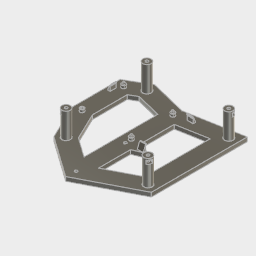
MPCNC Case 3 (Autodesk Fusion 360 design; units mm, degrees)
Autodesk Fusion 360 part; units mm, degrees
sketch "RAMBo" plane through (0, 0, 0) normal (0, 0, 1) x (1, 0, 0)
  line L0 (30.8759, -26.1352) -> (135.0159, -26.1352)
  line L1 (135.0159, -26.1352) -> (135.0159, 76.7348)
  line L2 (135.0159, 76.7348) -> (30.8759, 76.7348)
  line L3 (30.8759, 76.7348) -> (30.8759, -26.1352)
  line L4 (30.8759, 76.7348) -> (34.6859, 76.7348)
  line L5 (34.6859, 76.7348) -> (34.6859, 72.9248) construction
  line L6 (34.6859, 72.9248) -> (30.8759, 72.9248) construction
  line L7 (30.8759, 72.9248) -> (30.8759, 76.7348)
  line L8 (34.6859, 72.9248) -> (34.6859, -22.3252) construction
  line L9 (34.6859, -22.3252) -> (131.2059, -22.3252) construction
  line L10 (34.6859, 72.9248) -> (131.2059, 72.9248) construction
  circle A0 centre (34.6859, 72.9248) radius 1.625
  circle A1 centre (131.2059, 72.9248) radius 1.625
  circle A2 centre (34.6859, -22.3252) radius 1.625
  circle A3 centre (131.2059, -22.3252) radius 1.625
  line L11 (135.0159, -26.1352) -> (135.0159, 31.2053)
  line L12 (135.0159, -26.1352) -> (135.0159, 63.7808)
  line L13 (135.0159, 31.2053) -> (136.5659, 31.2053)
  line L14 (136.5659, 31.2053) -> (136.5659, 63.7808)
  line L15 (136.5659, 63.7808) -> (135.0159, 63.7808)
  line L16 (135.0159, 63.7808) -> (135.0159, 31.2053)
  line L17 (30.8759, -26.1352) -> (30.8759, 26.2523)
  line L18 (30.8759, -26.1352) -> (30.8759, 38.2538)
  line L19 (30.8759, 26.2523) -> (27.1959, 26.2523)
  line L20 (27.1959, 26.2523) -> (27.1959, 38.2538)
  line L21 (27.1959, 38.2538) -> (30.8759, 38.2538)
  line L22 (30.8759, 38.2538) -> (30.8759, 26.2523)
  dimension "d2" = 104.14
  dimension "d3" = 102.87
  dimension "d4" = 3.81
  dimension "d5" = 3.81
  dimension "d6" = 95.25
  dimension "d7" = 96.52
  dimension "d8" = 96.52
  dimension "d10" = 3.25
  dimension "d11" = 3.25
  dimension "d12" = 3.25
  dimension "d13" = 3.25
  dimension "d14" = 57.3405
  dimension "d15" = 89.916
  dimension "d16" = 1.55
  dimension "d17" = 52.3875
  dimension "d18" = 64.389
  dimension "d19" = 3.68
  measures "d2" distance of L0.start L0.end
  measures "d3" distance of L0.start L2.end
  measures "d4" distance of L2.end L6.end
  measures "d5" distance of L2.end L4.end
  measures "d6" distance of L5.end L8.end
  measures "d7" distance of L8.end L9.end
  measures "d8" distance of L5.end L10.end
  measures "d10" diameter of A0
  measures "d11" diameter of A1
  measures "d12" diameter of A2
  measures "d13" diameter of A3
  measures "d14" distance of L0.end L11.end
  measures "d15" distance of L0.end L12.end
  measures "d16" distance of L11.end L13.end
  measures "d17" distance of L0.start L17.end
  measures "d18" distance of L0.start L18.end
  measures "d19" distance of L17.end L19.end
sketch "RPi" plane through (0, 0, 0) normal (0, 0, 1) x (1, 0, 0)
  line L0 (17.3453, 10.3376) -> (17.3453, 13.8376) construction
  line L1 (17.3453, 13.8376) -> (13.8453, 13.8376) construction
  line L2 (16.8453, 10.3376) -> (16.8453, 13.3376) construction
  line L3 (16.8453, 13.3376) -> (13.8453, 13.3376) construction
  arc A0 (13.8453, 13.3376) -> (16.8453, 10.3376) centre (16.8453, 13.3376) ccw
  line L4 (16.8453, 66.3376) -> (16.8453, 63.3376) construction
  line L5 (16.8453, 63.3376) -> (13.8453, 63.3376) construction
  arc A1 (16.8453, 66.3376) -> (13.8453, 63.3376) centre (16.8453, 63.3376) ccw
  line L6 (95.8453, 66.3376) -> (95.8453, 63.3376) construction
  line L7 (95.8453, 63.3376) -> (98.8453, 63.3376) construction
  line L8 (95.8453, 10.3376) -> (95.8453, 13.3376) construction
  line L9 (95.8453, 13.3376) -> (98.8453, 13.3376) construction
  arc A2 (95.8453, 10.3376) -> (98.8453, 13.3376) centre (95.8453, 13.3376) ccw
  arc A3 (98.8453, 63.3376) -> (95.8453, 66.3376) centre (95.8453, 63.3376) ccw
  line L10 (17.3453, 66.3376) -> (17.3453, 62.8376) construction
  line L11 (17.3453, 62.8376) -> (13.8453, 62.8376) construction
  line L12 (17.3453, 62.8376) -> (75.3453, 62.8376) construction
  line L13 (17.3453, 13.8376) -> (75.3453, 13.8376) construction
  line L14 (75.3453, 13.8376) -> (75.3453, 10.3376) construction
  line L15 (98.8453, 13.3376) -> (98.8453, 63.3376)
  line L16 (95.8453, 66.3376) -> (16.8453, 66.3376)
  line L17 (13.8453, 63.3376) -> (13.8453, 13.3376)
  line L18 (16.8453, 10.3376) -> (95.8453, 10.3376)
  circle A4 centre (75.3453, 62.8376) radius 1.375
  circle A5 centre (75.3453, 13.8376) radius 1.375
  circle A6 centre (17.3453, 13.8376) radius 1.375
  circle A7 centre (17.3453, 62.8376) radius 1.375
  circle A8 centre (17.3453, 62.8376) radius 3.1 construction
  circle A9 centre (17.3453, 13.8376) radius 3.1 construction
  circle A10 centre (75.3453, 13.8376) radius 3.1 construction
  circle A11 centre (75.3453, 62.8376) radius 3.1 construction
  line L19 (13.8453, 13.3376) -> (24.4453, 13.3376) construction
  line L20 (24.4453, 13.3376) -> (24.4453, 10.3376) construction
  line L21 (20.9453, 11.3376) -> (27.9453, 11.3376)
  line L22 (27.9453, 11.3376) -> (27.9453, 9.3376)
  line L23 (27.9453, 9.3376) -> (20.9453, 9.3376)
  line L24 (20.9453, 9.3376) -> (20.9453, 11.3376)
  line L25 (20.9453, 11.3376) -> (27.9453, 9.3376) construction
  line L26 (27.9453, 11.3376) -> (20.9453, 9.3376) construction
  line L27 (13.8453, 13.3376) -> (45.8453, 13.3376) construction
  line L28 (45.8453, 13.3376) -> (45.8453, 10.3376) construction
  line L29 (38.5953, 8.3376) -> (53.0953, 8.3376)
  line L30 (53.0953, 8.3376) -> (53.0953, 12.3376)
  line L31 (53.0953, 12.3376) -> (38.5953, 12.3376)
  line L32 (38.5953, 12.3376) -> (38.5953, 8.3376)
  line L33 (38.5953, 8.3376) -> (53.0953, 12.3376) construction
  line L34 (53.0953, 8.3376) -> (38.5953, 12.3376) construction
  line L35 (13.8453, 13.3376) -> (67.3453, 13.3376) construction
  line L36 (67.3453, 13.3376) -> (67.3453, 10.3376) construction
  line L37 (65.3453, 12.3376) -> (69.3453, 12.3376)
  line L38 (69.3453, 12.3376) -> (69.3453, 8.3376)
  line L39 (69.3453, 8.3376) -> (65.3453, 8.3376)
  line L40 (65.3453, 8.3376) -> (65.3453, 12.3376)
  line L41 (65.3453, 12.3376) -> (69.3453, 8.3376) construction
  line L42 (69.3453, 12.3376) -> (65.3453, 8.3376) construction
  line L43 (16.8453, 10.3376) -> (16.8453, 38.3376) construction
  line L44 (16.8453, 38.3376) -> (13.8453, 38.3376) construction
  line L45 (16.8453, 43.8376) -> (10.8453, 43.8376)
  line L46 (10.8453, 43.8376) -> (10.8453, 32.8376)
  line L47 (10.8453, 32.8376) -> (16.8453, 32.8376)
  line L48 (16.8453, 32.8376) -> (16.8453, 43.8376)
  line L49 (16.8453, 43.8376) -> (10.8453, 32.8376) construction
  line L50 (10.8453, 43.8376) -> (16.8453, 32.8376) construction
  point P0 (24.4453, 10.3376)
  point P1 (45.8453, 10.3376)
  point P2 (67.3453, 10.3376)
  point P3 (13.8453, 38.3376)
  dimension "d83" = 10.6
  dimension "d85" = 2
  dimension "d86" = 7
  dimension "d87" = 32
  dimension "d88" = 14.5
  dimension "d89" = 4
  dimension "d90" = 53.5
  dimension "d91" = 4
  dimension "d92" = 4
  dimension "d127" = 28
  dimension "d128" = 11
  dimension "d129" = 6
  measures "d83" distance of L3.end L19.end
  measures "d85" distance of L21.end L22.end
  measures "d86" distance of L22.end L23.end
  measures "d87" distance of L3.end L27.end
  measures "d88" distance of L30.end L31.end
  measures "d89" distance of L29.end L30.end
  measures "d90" distance of L3.end L35.end
  measures "d91" distance of L37.end L38.end
  measures "d92" distance of L38.end L39.end
  measures "d127" distance of L2.start L43.end
  measures "d128" distance of L45.end L46.end
  measures "d129" distance of L46.end L47.end
sketch "TOBSUN Converter" plane through (0, 0, 0) normal (0, 0, 1) x (1, 0, 0)
  circle A0 centre (75.3453, 6.8376) radius 1.5
  circle A1 centre (75.3453, -51.1624) radius 1.5
  line L0 (56.3453, -47.1624) -> (109.3453, -47.1624)
  circle A2 centre (75.3453, -51.1624) radius 3.5
  line L1 (75.3453, 8.3376) -> (75.3453, 5.3376) construction
  line L2 (109.3453, 2.8376) -> (66.3453, 2.8376)
  line L3 (109.3453, 2.8376) -> (56.3453, 2.8376)
  line L4 (109.3453, -47.1624) -> (109.3453, 2.8376)
  line L5 (56.3453, 2.8376) -> (56.3453, -47.1624)
  line L6 (84.3453, -47.1624) -> (66.3453, -47.1624)
  line L7 (75.3453, 10.3376) -> (75.3453, 8.3376) construction
  line L8 (66.3453, 2.8376) -> (84.3453, 2.8376)
  line L9 (56.3453, 2.8376) -> (84.3453, 2.8376)
  line L10 (84.3453, 2.8376) -> (84.3453, -47.1624) construction
  line L11 (66.3453, 2.8376) -> (66.3453, -47.1624) construction
  line L12 (84.3453, -47.1624) -> (77.8106, -53.6469)
  line L13 (66.3453, -47.1624) -> (72.88, -53.6469)
  circle A3 centre (75.3453, 6.8376) radius 3.5
  line L14 (66.3453, 2.8376) -> (72.88, 9.322)
  line L15 (84.3453, 2.8376) -> (77.8106, 9.322)
  line L16 (109.3453, -47.1624) -> (109.3453, -22.1624)
  line L17 (109.3453, -22.1624) -> (138.1286, -22.1624) construction
  point P0 (109.3453, -47.1624)
  dimension "d55" = 53
  dimension "d56" = 50
  dimension "d57" = 28
  dimension "d58" = 43
  measures "d55" distance of P0 L0.start
  measures "d56" distance of L2.start P0
  measures "d57" distance of L3.end L8.end
  measures "d58" distance of L2.start L2.end
sketch "Case Sketch" plane through (0, 0, 0) normal (0, 0, 1) x (1, 0, 0)
  circle A0 centre (75.3453, 6.8376) radius 1.625
  circle A1 centre (75.3453, -51.1624) radius 1.625
  circle A2 centre (75.3453, 6.8376) radius 3
  circle A3 centre (75.3453, -51.1624) radius 3
  circle A4 centre (75.3453, 13.8376) radius 1.125
  circle A5 centre (17.3453, 13.8376) radius 1.375
  circle A6 centre (75.3453, 62.8376) radius 1.125
  circle A7 centre (17.3453, 62.8376) radius 1.125
  circle A8 centre (75.3453, 13.8376) radius 2.5
  circle A9 centre (75.3453, 62.8376) radius 2.5
  circle A10 centre (17.3453, 62.8376) radius 2.5
  circle A11 centre (17.3453, 13.8376) radius 2.5
  circle A12 centre (34.6859, 72.9248) radius 1.625
  circle A13 centre (131.2059, 72.9248) radius 1.625
  circle A14 centre (34.6859, -22.3252) radius 1.625
  circle A15 centre (131.2059, -22.3252) radius 1.625
  circle A16 centre (34.6859, 72.9248) radius 5
  circle A17 centre (131.2059, 72.9248) radius 5
  circle A18 centre (131.2059, -22.3252) radius 5
  circle A19 centre (34.6859, -22.3252) radius 5
  line L0 (17.3453, 13.8376) -> (17.3453, 62.8376) construction
  line L1 (17.3453, 62.8376) -> (34.6859, 72.9248) construction
  line L2 (34.6859, 72.9248) -> (75.3453, 62.8376) construction
  line L3 (75.3453, 62.8376) -> (131.2059, 72.9248) construction
  line L4 (131.2059, 72.9248) -> (131.2059, -22.3252) construction
  line L5 (131.2059, -22.3252) -> (75.3453, -51.1624) construction
  line L6 (75.3453, -51.1624) -> (34.6859, -22.3252) construction
  line L7 (34.6859, -22.3252) -> (17.3453, 13.8376) construction
  line L8 (75.3453, 62.8376) -> (75.3453, 13.8376) construction
  line L9 (75.3453, 13.8376) -> (75.3453, 6.8376)
  line L10 (75.3453, 6.8376) -> (75.3453, -51.1624) construction
  line L11 (27.3453, 16.1112) -> (27.3453, 57.0858)
  line L12 (27.3453, 57.0858) -> (36.2112, 62.2433)
  line L13 (121.2059, 60.9573) -> (121.2059, -16.2336)
  line L14 (42.5832, -15.6665) -> (27.3453, 16.1112)
  line L15 (7.3453, 11.5639) -> (7.3453, 68.5893)
  line L16 (7.3453, 68.5893) -> (33.1605, 83.6064)
  line L17 (33.1605, 83.6064) -> (75.6752, 73.0589)
  line L18 (75.6752, 73.0589) -> (141.2059, 84.8924)
  line L19 (141.2059, 84.8924) -> (141.2059, -28.4167)
  line L20 (141.2059, -28.4167) -> (74.5245, -62.8401)
  line L21 (74.5245, -62.8401) -> (26.7886, -28.9839)
  line L22 (26.7886, -28.9839) -> (7.3453, 11.5639)
  line L23 (65.3453, 13.8376) -> (65.3453, 6.8376)
  line L24 (65.3453, 6.8376) -> (65.3453, -31.8103)
  line L25 (65.3453, -31.8103) -> (42.5832, -15.6665)
  line L26 (85.3453, 13.8376) -> (85.3453, 6.8376)
  line L27 (121.2059, -16.2336) -> (85.3453, -34.7462)
  line L28 (42.5832, -15.6665) -> (65.3453, -31.8103)
  line L29 (42.5832, -15.6665) -> (27.3453, 16.1112)
  line L30 (65.3453, -31.8103) -> (65.3453, 55.0153)
  line L31 (121.2059, 60.9573) -> (85.3453, 54.4816)
  line L32 (36.2112, 62.2433) -> (65.3453, 55.0153)
  line L33 (85.3453, -34.7462) -> (85.3453, 54.4816)
  line L34 (34.6859, 72.9248) -> (45.0296, 72.9248) construction
  line L35 (34.6859, -22.3252) -> (39.6859, -22.3252) construction
  line L36 (37.5359, -20.6797) -> (34.6859, -19.0343)
  line L37 (34.6859, -19.0343) -> (31.8359, -20.6797)
  line L38 (31.8359, -20.6797) -> (31.8359, -23.9706)
  line L39 (31.8359, -23.9706) -> (34.6859, -25.6161)
  line L40 (34.6859, -25.6161) -> (37.5359, -23.9706)
  line L41 (37.5359, -23.9706) -> (37.5359, -20.6797)
  line L42 (31.8359, -20.6797) -> (29.703, -21.9111)
  line L43 (34.6859, -25.6161) -> (32.553, -26.8474)
  line L44 (128.3559, -23.9706) -> (131.2059, -25.6161)
  line L45 (131.2059, -25.6161) -> (134.0559, -23.9706)
  line L46 (134.0559, -23.9706) -> (134.0559, -20.6797)
  line L47 (134.0559, -20.6797) -> (131.2059, -19.0343)
  line L48 (131.2059, -19.0343) -> (128.3559, -20.6797)
  line L49 (128.3559, -20.6797) -> (128.3559, -23.9706)
  line L50 (131.2059, -25.6161) -> (133.3387, -26.8474)
  line L51 (134.0559, -20.6797) -> (136.1887, -21.9111)
  line L52 (134.0559, 74.5703) -> (131.2059, 76.2157)
  line L53 (131.2059, 76.2157) -> (128.3559, 74.5703)
  line L54 (128.3559, 74.5703) -> (128.3559, 71.2794)
  line L55 (128.3559, 71.2794) -> (131.2059, 69.6339)
  line L56 (131.2059, 69.6339) -> (134.0559, 71.2794)
  line L57 (134.0559, 71.2794) -> (134.0559, 74.5703)
  line L58 (131.2059, 76.2157) -> (133.3387, 77.4471)
  line L59 (134.0559, 71.2794) -> (136.1887, 72.5108)
  line L60 (31.8359, 71.2794) -> (34.6859, 69.6339)
  line L61 (34.6859, 69.6339) -> (37.5359, 71.2794)
  line L62 (37.5359, 71.2794) -> (37.5359, 74.5703)
  line L63 (37.5359, 74.5703) -> (34.6859, 76.2157)
  line L64 (34.6859, 76.2157) -> (31.8359, 74.5703)
  line L65 (31.8359, 74.5703) -> (31.8359, 71.2794)
  line L66 (34.6859, 76.2157) -> (32.553, 77.4471)
  line L67 (31.8359, 71.2794) -> (29.703, 72.5108)
  point P0 (75.3453, 6.8376)
  point P1 (75.3453, -51.1624)
  point P2 (75.3453, 13.8376)
  point P3 (17.3453, 13.8376)
  point P4 (75.3453, 62.8376)
  point P5 (17.3453, 62.8376)
  point P6 (34.6859, 72.9248)
  point P7 (131.2059, 72.9248)
  point P8 (34.6859, -22.3252)
  point P9 (131.2059, -22.3252)
  point P10 (34.6859, -22.3252)
  point P11 (131.2059, -22.3252)
  point P12 (131.2059, 72.9248)
  point P13 (34.6859, 72.9248)
  dimension "d70" = 3.25
  dimension "d71" = 3.25
  dimension "d72" = 6
  dimension "d73" = 6
  dimension "d74" = 2.25
  dimension "d76" = 2.75
  dimension "d77" = 2.25
  dimension "d78" = 2.25
  dimension "d79" = 5
  dimension "d80" = 5
  dimension "d81" = 5
  dimension "d82" = 5
  dimension "d93" = 3.25
  dimension "d94" = 3.25
  dimension "d95" = 3.25
  dimension "d96" = 3.25
  dimension "d97" = 10
  dimension "d98" = 10
  dimension "d99" = 10
  dimension "d100" = 10
  dimension "d102" = 10
  dimension "d119" = 2.85
  dimension "d120" = 2.85
  dimension "d121" = 2.85
  dimension "d122" = 2.85
  measures "d70" diameter of A0
  measures "d71" diameter of A1
  measures "d72" diameter of A2
  measures "d73" diameter of A3
  measures "d74" diameter of A4
  measures "d76" diameter of A5
  measures "d77" diameter of A6
  measures "d78" diameter of A7
  measures "d79" diameter of A8
  measures "d80" diameter of A9
  measures "d81" diameter of A10
  measures "d82" diameter of A11
  measures "d93" diameter of A12
  measures "d94" diameter of A13
  measures "d95" diameter of A14
  measures "d96" diameter of A15
  measures "d97" diameter of A16
  measures "d98" diameter of A17
  measures "d99" diameter of A18
  measures "d100" diameter of A19
  measures "d119" distance of P10 L41
  measures "d120" distance of P11 L49
  measures "d121" distance of P12 L57
  measures "d122" distance of P13 L65
extrude "Extrude1" add sketch "Case Sketch" against normal blind 5 contours A0 | A1 | A2 | A3 | A4 | A5 | A6 | A7 | A8 | A9 | A10 | A11 | A12 | A13 | A14 | A15 | A16 L60 L61 L62 L63 L66 L67 | A16 L64 L65 L66 L67 | L60 L61 L62 L63 L64 L65 | A17 L52 L57 L58 L59 | A17 L53 L54 L55 L56 L58 L59 | L52 L53 L54 L55 L56 L57 | A18 L45 L46 L50 L51 | A18 L44 L47 L48 L49 L50 L51 | L44 L45 L46 L47 L48 L49 | A19 L36 L37 L40 L41 L42 L43 | A19 L38 L39 L42 L43 | L36 L37 L38 L39 L40 L41 | L15 L16 L17 L18 L19 L20 L21 L22 makes body 1
extrude "Extrude2" cut sketch "Case Sketch" against normal through all contours A0 | A1 | A2 | A3 bodies 1
extrude "Extrude3" add sketch "Case Sketch" against normal blind 2 contours A2 | A3 bodies 1
extrude "Extrude4" cut sketch "Case Sketch" against normal through all contours A12 | A13 | A14 | A15 bodies 1
extrude "Extrude5" add sketch "Case Sketch" along normal blind 30 contours A16 L60 L61 L62 L63 L66 L67 | A16 L64 L65 L66 L67 | L60 L61 L62 L63 L64 L65 | A17 L52 L57 L58 L59 | A17 L53 L54 L55 L56 L58 L59 | L52 L53 L54 L55 L56 L57 | A18 L45 L46 L50 L51 | A18 L44 L47 L48 L49 L50 L51 | L44 L45 L46 L47 L48 L49 | A19 L36 L37 L40 L41 L42 L43 | A19 L38 L39 L42 L43 | L36 L37 L38 L39 L40 L41 bodies 1
extrude "Extrude6" add sketch "Case Sketch" along normal blind 3 contours A8 | A9 | A10 | A11 bodies 1
extrude "Extrude7" add sketch "Case Sketch" along normal blind 5 separate body contours A4 | A6 | A7 makes body 2 at (16.2882, 62.4528, 3.3333) makes body 3 at (74.2882, 62.4528, 3.3333) makes body 4 at (74.5598, 13.0322, 3.3333)
combine "Combine1" operation add target body 1 tool bodies 2 4 3
extrude "Extrude8" cut sketch "Case Sketch" along normal blind 28 contours A16 L64 L65 L66 L67 | L60 L61 L62 L63 L64 L65 | A17 L52 L57 L58 L59 | L52 L53 L54 L55 L56 L57 | A18 L45 L46 L50 L51 | L44 L45 L46 L47 L48 L49 | A19 L38 L39 L42 L43 | L36 L37 L38 L39 L40 L41 bodies 1
extrude "Extrude9" add sketch "Case Sketch" along normal blind 24 contours A16 L60 L61 L62 L63 L66 L67 | A16 L64 L65 L66 L67 | L60 L61 L62 L63 L64 L65 | A17 L52 L57 L58 L59 | A17 L53 L54 L55 L56 L58 L59 | L52 L53 L54 L55 L56 L57 | A18 L45 L46 L50 L51 | A18 L44 L47 L48 L49 L50 L51 | L44 L45 L46 L47 L48 L49 | A19 L36 L37 L40 L41 L42 L43 | A19 L38 L39 L42 L43 | L36 L37 L38 L39 L40 L41 bodies 1
sketch "RPi Latch" plane through (0, 50.4214, 0) normal (0, -1, 0) x (1, 0, 0)
  line L0 (10.8453, 0) -> (13.8453, 0)
  line L1 (13.8453, 0) -> (13.8453, 7)
  line L2 (13.8453, 7) -> (14.8453, 7)
  line L3 (13.8453, 7) -> (13.8453, 5)
  line L4 (14.8453, 7) -> (13.8453, 5)
  line L5 (13.8453, 7) -> (10.8453, 0)
  line L6 (13.8453, 5) -> (13.8453, 0)
  dimension "d135" = 1
  dimension "d136" = 2
  measures "d135" distance of L1.end L2.end
  measures "d136" distance of L1.end L3.end
extrude "Extrude10" add sketch "RPi Latch" against normal blind 7 separate body makes body 5
copy_body "CopyPasteBodies1" bodies 5 makes body 6
move_body "Move1" bodies 6 to x (1, 0, 0) y (0, 1, 0) z (0, 0, 1) at (76, 16, 0)
move_body "Move2" bodies 6 to x (0, -1, 0) y (1, 0, 0) z (0, 0, 1) at (0, 0, 0)
move_body "Move3" bodies 6 to x (1, 0, 0) y (0, 1, 0) z (0, 0, 1) at (21, 156.5, 0)
move_body "Move4" bodies 6 to x (1, 0, 0) y (0, 1, 0) z (0, 0, 1) at (1.4239, -0.3171, 0)
copy_body "CopyPasteBodies2" bodies 6 makes body 7
move_body "Move5" bodies 7 to x (1, 0, 0) y (0, 1, 0) z (0, 0, 1) at (0, -218.4738, 94.076)
move_body "Move6" bodies 7 to x (-1, 0, 0) y (0, -1, 0) z (0, 0, 1) at (0, 0, 0)
move_body "Move7" bodies 7 to x (1, 0, 0) y (0, 1, 0) z (0, 0, 1) at (210, 0, -168)
move_body "Move8" bodies 7 to x (1, 0, 0) y (0, 1, 0) z (0, 0, 1) at (-25.3094, -141.7987, 73.924)
sketch "Inside Latch Base" plane through (0, 0, 0) normal (0, 0, 1) x (1, 0, 0)
  line L0 (88.8453, 11.3376) -> (95.8453, 11.3376)
  line L1 (95.8453, 11.3376) -> (95.8453, 7.3376)
  line L2 (95.8453, 7.3376) -> (88.8453, 7.3376)
  line L3 (88.8453, 7.3376) -> (88.8453, 11.3376)
  line L4 (83.8453, 2.3376) -> (83.8453, 16.3376)
  line L5 (83.8453, 16.3376) -> (95.8453, 11.3376)
  line L6 (83.8453, 2.3376) -> (95.8453, 7.3376)
  point P0 (88.8453, 11.3376)
  point P1 (95.8453, 7.3376)
extrude "Extrude11" add sketch "Inside Latch Base" against normal blind 5 bodies 1
equation "d4 = ( 4050 mil - 3750 mil ) / 2"
equation "d5 = ( 4100 mil - 3800 mil ) / 2"
equation "d11 = ( 1.625 * 2 ) * 1 mm"
equation "d70 = ( 1.625 * 2 ) * 1 mm"
equation "d71 = ( 1.625 * 2 ) * 1 mm"
equation "d125 = 28 mm - 4 mm"
named bodies: "Case", "RPi Latch Front", "RPi Latch Outside", "RPi Latch Inside"
